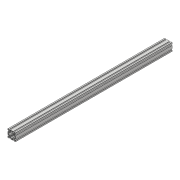
# Autodesk Inventor part: HFS5-4040-800
Saved by Autodesk Inventor 2018 (Build 220112000, 112)
## iProperties
Created: 2018-01-07
Part Number: HFS5-4040-800
Material: Generic
Document SubType Name: Modeling
Designer: sawaiz
Density: 1 g/cm^3
Appearance: Default
Author: sawaiz
Autodesk Inventor part; units mm, degrees
ref_plane "YZ Plane" through (0, 0, 0) normal (1, 0, 0) x (0, 1, 0)
ref_plane "XZ Plane" through (0, 0, 0) normal (0, 1, 0) x (-1, 0, 0)
ref_plane "XY Plane" through (0, 0, 0) normal (0, 0, 1) x (1, 0, 0)
sketch "Sketch1" plane through (0, 0, 0) normal (0, 1, 0) x (-1, 0, 0)
  line L0 (-20, 7) -> (-20, -7)
  line L1 (-20, -7) -> (-18, -7)
  line L2 (-18, -7) -> (-18, -4)
  line L3 (-18, -4) -> (-17.0607, -4)
  line L4 (-17.0607, -4) -> (-14, -7.0607)
  line L5 (-14, -7.0607) -> (-14, -9.3464)
  arc A0 (-14, -9.3464) -> (-13.933, -9.5964) centre (-13.5, -9.3464) ccw
  line L6 (-13.933, -9.5964) -> (-13.7, -10)
  line L7 (-13.7, -10) -> (-13.933, -10.4036)
  arc A1 (-13.933, -10.4036) -> (-13.933, -10.9036) centre (-13.5, -10.6536) ccw
  line L8 (-13.933, -10.9036) -> (-13.751, -11.2189)
  line L9 (-13.751, -11.2189) -> (-14, -12.5)
  line L10 (-14, -12.5) -> (-14, -12.9393)
  line L11 (-14, -12.9393) -> (-17.0607, -16)
  line L12 (-17.0607, -16) -> (-18, -16)
  line L13 (-18, -16) -> (-18, -13)
  line L14 (-18, -13) -> (-20, -13)
  line L15 (-20, -13) -> (-20, -19)
  arc A2 (-20, -19) -> (-19, -20) centre (-19, -19) ccw
  line L16 (-19, -20) -> (-13, -20)
  line L17 (-13, -20) -> (-13, -18)
  line L18 (-13, -18) -> (-16, -18)
  line L19 (-16, -18) -> (-16, -17.0607)
  line L20 (-16, -17.0607) -> (-12.9393, -14)
  line L21 (-12.9393, -14) -> (-10.6536, -14)
  arc A3 (-10.6536, -14) -> (-10.4036, -13.933) centre (-10.6536, -13.5) ccw
  line L22 (-10.4036, -13.933) -> (-10, -13.7)
  line L23 (-10, -13.7) -> (-9.5964, -13.933)
  arc A4 (-9.5964, -13.933) -> (-9.0964, -13.933) centre (-9.3464, -13.5) ccw
  line L24 (-9.0964, -13.933) -> (-8.7811, -13.751)
  line L25 (-8.7811, -13.751) -> (-7.5, -14)
  line L26 (-7.5, -14) -> (-7.0607, -14)
  line L27 (-7.0607, -14) -> (-4, -17.0607)
  line L28 (-4, -17.0607) -> (-4, -18)
  line L29 (-4, -18) -> (-7, -18)
  line L30 (-7, -18) -> (-7, -20)
  line L31 (-7, -20) -> (7, -20)
  line L32 (7, -20) -> (7, -18)
  line L33 (7, -18) -> (4, -18)
  line L34 (4, -18) -> (4, -17.0607)
  line L35 (4, -17.0607) -> (7.0607, -14)
  line L36 (7.0607, -14) -> (9.3464, -14)
  arc A5 (9.3464, -14) -> (9.5964, -13.933) centre (9.3464, -13.5) ccw
  line L37 (9.5964, -13.933) -> (10, -13.7)
  line L38 (10, -13.7) -> (10.4036, -13.933)
  arc A6 (10.4036, -13.933) -> (10.9036, -13.933) centre (10.6536, -13.5) ccw
  line L39 (10.9036, -13.933) -> (11.2189, -13.751)
  line L40 (11.2189, -13.751) -> (12.5, -14)
  line L41 (12.5, -14) -> (12.9393, -14)
  line L42 (12.9393, -14) -> (16, -17.0607)
  line L43 (16, -17.0607) -> (16, -18)
  line L44 (16, -18) -> (13, -18)
  line L45 (13, -18) -> (13, -20)
  line L46 (13, -20) -> (19, -20)
  arc A7 (19, -20) -> (20, -19) centre (19, -19) ccw
  line L47 (20, -19) -> (20, -13)
  line L48 (20, -13) -> (18, -13)
  line L49 (18, -13) -> (18, -16)
  line L50 (18, -16) -> (17.0607, -16)
  line L51 (17.0607, -16) -> (14, -12.9393)
  line L52 (14, -12.9393) -> (14, -10.6536)
  arc A8 (14, -10.6536) -> (13.933, -10.4036) centre (13.5, -10.6536) ccw
  line L53 (13.933, -10.4036) -> (13.7, -10)
  line L54 (13.7, -10) -> (13.933, -9.5964)
  arc A9 (13.933, -9.5964) -> (13.933, -9.0964) centre (13.5, -9.3464) ccw
  line L55 (13.933, -9.0964) -> (13.751, -8.7811)
  line L56 (13.751, -8.7811) -> (14, -7.5)
  line L57 (14, -7.5) -> (14, -7.0607)
  line L58 (14, -7.0607) -> (17.0607, -4)
  line L59 (17.0607, -4) -> (18, -4)
  line L60 (18, -4) -> (18, -7)
  line L61 (18, -7) -> (20, -7)
  line L62 (20, -7) -> (20, 7)
  line L63 (20, 7) -> (18, 7)
  line L64 (18, 7) -> (18, 4)
  line L65 (18, 4) -> (17.0607, 4)
  line L66 (17.0607, 4) -> (14, 7.0607)
  line L67 (14, 7.0607) -> (14, 9.3464)
  arc A10 (14, 9.3464) -> (13.933, 9.5964) centre (13.5, 9.3464) ccw
  line L68 (13.933, 9.5964) -> (13.7, 10)
  line L69 (13.7, 10) -> (13.933, 10.4036)
  arc A11 (13.933, 10.4036) -> (13.933, 10.9036) centre (13.5, 10.6536) ccw
  line L70 (13.933, 10.9036) -> (13.751, 11.2189)
  line L71 (13.751, 11.2189) -> (14, 12.5)
  line L72 (14, 12.5) -> (14, 12.9393)
  line L73 (14, 12.9393) -> (17.0607, 16)
  line L74 (17.0607, 16) -> (18, 16)
  line L75 (18, 16) -> (18, 13)
  line L76 (18, 13) -> (20, 13)
  line L77 (20, 13) -> (20, 19)
  arc A12 (20, 19) -> (19, 20) centre (19, 19) ccw
  line L78 (19, 20) -> (13, 20)
  line L79 (13, 20) -> (13, 18)
  line L80 (13, 18) -> (16, 18)
  line L81 (16, 18) -> (16, 17.0607)
  line L82 (16, 17.0607) -> (12.9393, 14)
  line L83 (12.9393, 14) -> (10.6536, 14)
  arc A13 (10.6536, 14) -> (10.4036, 13.933) centre (10.6536, 13.5) ccw
  line L84 (10.4036, 13.933) -> (10, 13.7)
  line L85 (10, 13.7) -> (9.5964, 13.933)
  arc A14 (9.5964, 13.933) -> (9.0964, 13.933) centre (9.3464, 13.5) ccw
  line L86 (9.0964, 13.933) -> (8.7811, 13.751)
  line L87 (8.7811, 13.751) -> (7.5, 14)
  line L88 (7.5, 14) -> (7.0607, 14)
  line L89 (7.0607, 14) -> (4, 17.0607)
  line L90 (4, 17.0607) -> (4, 18)
  line L91 (4, 18) -> (7, 18)
  line L92 (7, 18) -> (7, 20)
  line L93 (7, 20) -> (-7, 20)
  line L94 (-7, 20) -> (-7, 18)
  line L95 (-7, 18) -> (-4, 18)
  line L96 (-4, 18) -> (-4, 17.0607)
  line L97 (-4, 17.0607) -> (-7.0607, 14)
  line L98 (-7.0607, 14) -> (-9.3464, 14)
  arc A15 (-9.3464, 14) -> (-9.5964, 13.933) centre (-9.3464, 13.5) ccw
  line L99 (-9.5964, 13.933) -> (-10, 13.7)
  line L100 (-10, 13.7) -> (-10.4036, 13.933)
  arc A16 (-10.4036, 13.933) -> (-10.9036, 13.933) centre (-10.6536, 13.5) ccw
  line L101 (-10.9036, 13.933) -> (-11.2189, 13.751)
  line L102 (-11.2189, 13.751) -> (-12.5, 14)
  line L103 (-12.5, 14) -> (-12.9393, 14)
  line L104 (-12.9393, 14) -> (-16, 17.0607)
  line L105 (-16, 17.0607) -> (-16, 18)
  line L106 (-16, 18) -> (-13, 18)
  line L107 (-13, 18) -> (-13, 20)
  line L108 (-13, 20) -> (-19, 20)
  arc A17 (-19, 20) -> (-20, 19) centre (-19, 19) ccw
  line L109 (-20, 19) -> (-20, 13)
  line L110 (-20, 13) -> (-18, 13)
  line L111 (-18, 13) -> (-18, 16)
  line L112 (-18, 16) -> (-17.0607, 16)
  line L113 (-17.0607, 16) -> (-14, 12.9393)
  line L114 (-14, 12.9393) -> (-14, 10.6536)
  arc A18 (-14, 10.6536) -> (-13.933, 10.4036) centre (-13.5, 10.6536) ccw
  line L115 (-13.933, 10.4036) -> (-13.7, 10)
  line L116 (-13.7, 10) -> (-13.933, 9.5964)
  arc A19 (-13.933, 9.5964) -> (-13.933, 9.0964) centre (-13.5, 9.3464) ccw
  line L117 (-13.933, 9.0964) -> (-13.751, 8.7811)
  line L118 (-13.751, 8.7811) -> (-14, 7.5)
  line L119 (-14, 7.5) -> (-14, 7.0607)
  line L120 (-14, 7.0607) -> (-17.0607, 4)
  line L121 (-17.0607, 4) -> (-18, 4)
  line L122 (-18, 4) -> (-18, 7)
  line L123 (-18, 7) -> (-20, 7)
  line L124 (18, -2) -> (18, 2)
  line L125 (-16.9393, 2) -> (-18, 2)
  line L126 (-12.9393, 6) -> (-16.9393, 2)
  line L127 (-8.6667, 6) -> (-12.9393, 6)
  line L128 (-9.3359, 8.0078) -> (-8.6667, 6)
  arc A20 (-8.0078, 9.3359) -> (-9.3359, 8.0078) centre (-10, 10) ccw
  line L129 (-6, 8.6667) -> (-8.0078, 9.3359)
  line L130 (-6, 12.9393) -> (-6, 8.6667)
  line L131 (-2, 16.9393) -> (-6, 12.9393)
  line L132 (-2, 18) -> (-2, 16.9393)
  line L133 (2, 18) -> (-2, 18)
  line L134 (2, 16.9393) -> (2, 18)
  line L135 (6, 12.9393) -> (2, 16.9393)
  line L136 (6, 8.6667) -> (6, 12.9393)
  line L137 (8.0078, 9.3359) -> (6, 8.6667)
  arc A21 (9.3359, 8.0078) -> (8.0078, 9.3359) centre (10, 10) ccw
  line L138 (8.6667, 6) -> (9.3359, 8.0078)
  line L139 (12.9393, 6) -> (8.6667, 6)
  line L140 (16.9393, 2) -> (12.9393, 6)
  line L141 (18, 2) -> (16.9393, 2)
  line L142 (16.9393, -2) -> (18, -2)
  line L143 (12.9393, -6) -> (16.9393, -2)
  line L144 (8.6667, -6) -> (12.9393, -6)
  line L145 (9.3359, -8.0078) -> (8.6667, -6)
  arc A22 (8.0078, -9.3359) -> (9.3359, -8.0078) centre (10, -10) ccw
  line L146 (6, -8.6667) -> (8.0078, -9.3359)
  line L147 (6, -12.9393) -> (6, -8.6667)
  line L148 (2, -16.9393) -> (6, -12.9393)
  line L149 (2, -18) -> (2, -16.9393)
  line L150 (-2, -18) -> (2, -18)
  line L151 (-2, -16.9393) -> (-2, -18)
  line L152 (-6, -12.9393) -> (-2, -16.9393)
  line L153 (-6, -8.6667) -> (-6, -12.9393)
  line L154 (-8.0078, -9.3359) -> (-6, -8.6667)
  arc A23 (-9.3359, -8.0078) -> (-8.0078, -9.3359) centre (-10, -10) ccw
  line L155 (-8.6667, -6) -> (-9.3359, -8.0078)
  line L156 (-12.9393, -6) -> (-8.6667, -6)
  line L157 (-16.9393, -2) -> (-12.9393, -6)
  line L158 (-18, -2) -> (-16.9393, -2)
  line L159 (-18, 2) -> (-18, -2)
  line L160 (10, -10) -> (-10, 10) construction
  point P0 (0, 0)
  point P1 (0, 0)
  constraints: 322 end point, 48 point on circle, 24 centre point, 1 midpoint
extrude "Extrusion1" add sketch "Sketch1" along normal mid plane 800
body "Solid1"
